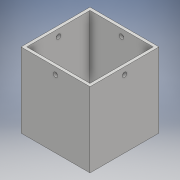
# Autodesk Inventor part: Box
Saved by Autodesk Inventor 2017 (Build 210142000, 142)
## iProperties
Created: 2017-02-24
Part Number: Box
Material: Generic
Document SubType Name: Modeling
Designer: aribu
Density: 1 g/cm^3
Appearance: Default
Author: aribu
Autodesk Inventor part; units mm, degrees
ref_plane "YZ Plane" through (0, 0, 0) normal (1, 0, 0) x (0, 1, 0)
ref_plane "XZ Plane" through (0, 0, 0) normal (0, 1, 0) x (-1, 0, 0)
ref_plane "XY Plane" through (0, 0, 0) normal (0, 0, 1) x (1, 0, 0)
sketch "Sketch1" plane through (0, 0, 0) normal (0, 0, 1) x (1, 0, 0)
  line L0 (-55, 55) -> (55, 55)
  line L1 (55, 55) -> (55, -55)
  line L2 (55, -55) -> (-55, -55)
  line L3 (-55, -55) -> (-55, 55)
  line L4 (-60, 60) -> (60, 60)
  line L5 (60, 60) -> (60, -60)
  line L6 (60, -60) -> (-60, -60)
  line L7 (-60, -60) -> (-60, 60)
  point P0 (0, 0)
  dimension "d0" = 110
  dimension "d1" = 110
  dimension "d2" = 55
  dimension "d3" = 55
  dimension "d4" = 5
  dimension "d5" = 5
  dimension "d6" = 5
  dimension "d7" = 5
  constraints: 16 end point, 4 parallel, 2 horizontal, 2 perpendicular
  measures "d0" distance of L0.start L0.end
  measures "d1" distance of L0.end L1.end
  measures "d2" distance from line of point (0, 0) L0
  measures "d3" distance from line of L1 point (0, 0)
  measures "d4" distance between parallel lines of L0 L4
  measures "d5" distance between parallel lines of L3 L7
  measures "d6" distance between parallel lines of L6 L2
  measures "d7" distance between parallel lines of L5 L1
extrude "Extrusion1" add sketch "Sketch1" along normal blind 120
sketch "Sketch2" plane through (0, 0, 0) normal (0, 0, -1) x (-1, 0, 0)
  line L0 (60, 60) -> (60, -60) projected
  line L1 (-60, 60) -> (60, 60)
  line L2 (60, 60) -> (60, -60)
  line L3 (60, -60) -> (-60, -60)
  line L4 (-60, -60) -> (-60, 60)
  point P0 (0, 0)
  constraints: 8 end point, 2 parallel, 1 horizontal, 1 perpendicular
extrude "Extrusion2" add sketch "Sketch2" along normal blind 10
sketch "Sketch3" plane through (-60, -60, 120) normal (0, -1, 0) x (1, 0, 0)
  circle A0 centre (60, -12) radius 4
  line L0 (0, 0) -> (120, 0) projected
  line L1 (120, 0) -> (120, -130) projected
  point P0 (60, -120)
  dimension "d12" = 8
  dimension "d13" = 12
  dimension "d14" = 60
  constraints: 1 centre point
  measures "d12" diameter of A0
  measures "d13" distance from line of L0 A0.centre
  measures "d14" distance from line of L1 A0.centre
sketch "Sketch4" plane through (60, -60, 120) normal (1, 0, 0) x (0, 0, -1)
  circle A0 centre (12, 60) radius 4
  line L0 (0, 0) -> (0, 120) projected
  line L1 (0, 120) -> (130, 120) projected
  point P0 (60, -120)
  dimension "d15" = 8
  dimension "d18" = 12
  dimension "d19" = 60
  constraints: 1 centre point
  measures "d15" diameter of A0
  measures "d18" distance from line of A0.centre L0
  measures "d19" distance from line of L1 A0.centre
extrude "Extrusion3" cut sketch "Sketch4" against normal blind 120
extrude "Extrusion4" cut sketch "Sketch3" against normal blind 120
equation "\"d1\" = d0"
equation "\"d2\" = 0.5 * d0"
equation "\"d3\" = 0.5 * d0"
equation "\"d5\" = d4"
equation "\"d6\" = d4"
equation "\"d7\" = d4"
body "Solid1"
